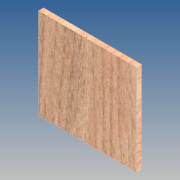
# Autodesk Inventor part: 2203_Housing Back
Saved by Autodesk Inventor 2020 (Build 240168000, 168)
## iProperties
Created: 2019-11-08
Part Number: 2203_Housing Back
Material: Wood (Birch)
Document SubType Name: Modeling
Designer: RFLab
Density: 0.55 g/cm^3
Appearance: Birch - Natural Polished
Author: RFLab
Autodesk Inventor part; units mm, degrees
ref_plane "YZ Plane" through (0, 0, 0) normal (1, 0, 0) x (0, 1, 0)
ref_plane "XZ Plane" through (0, 0, 0) normal (0, 1, 0) x (-1, 0, 0)
ref_plane "XY Plane" through (0, 0, 0) normal (0, 0, 1) x (1, 0, 0)
sketch "Sketch1" plane through (0, 0, 0) normal (0, 0, 1) x (1, 0, 0)
  line L0 (-61.15, 56.825) -> (61.15, 56.825)
  line L1 (61.15, 56.825) -> (61.15, -56.825)
  line L2 (61.15, -56.825) -> (-61.15, -56.825)
  line L3 (-61.15, -56.825) -> (-61.15, 56.825)
  point P0 (0, 0)
  dimension "d0" = 122.3
  dimension "d1" = 113.65
  dimension "d2" = 56.825
  dimension "d3" = 61.15
  constraints: 8 end point, 2 parallel, 1 horizontal, 1 perpendicular
  measures "d0" distance of L1.end L2.end
  measures "d1" distance of L0.end L1.end
  measures "d2" distance from line of point (0, 0) L2
  measures "d3" distance from line of L3 point (0, 0)
extrude "Extrusion1" add sketch "Sketch1" along normal blind 6.35
equation "\"d2\" = 0.5 * d1"
equation "\"d3\" = 0.5 * d0"
body "Solid1"
